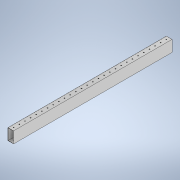
# Autodesk Inventor part: 28in OChannel 1x2
Saved by Autodesk Inventor 2020 (Build 240168000, 168)
## iProperties
Created: 2021-02-04
Part Number: 28in OChannel 1x2
Material: Aluminum 6061-AHC
Document SubType Name: Modeling
Designer: sidsa
Density: 2.7 g/cm^3
Appearance: Aluminum - Dark
Author: sidsa
Autodesk Inventor part; units mm, degrees
ref_plane "YZ Plane" through (0, 0, 0) normal (1, 0, 0) x (0, 1, 0)
ref_plane "XZ Plane" through (0, 0, 0) normal (0, 1, 0) x (-1, 0, 0)
ref_plane "XY Plane" through (0, 0, 0) normal (0, 0, 1) x (1, 0, 0)
sketch "Sketch1" plane through (0, 0, 0) normal (0, 0, 1) x (1, 0, 0)
  line L0 (0, 0) -> (25.4, 0)
  line L1 (25.4, 0) -> (25.4, 50.8)
  line L2 (25.4, 50.8) -> (0, 50.8)
  line L3 (0, 50.8) -> (0, 0)
  line L4 (24.384, 49.784) -> (24.384, 1.016)
  line L5 (24.384, 1.016) -> (1.016, 1.016)
  line L6 (1.016, 1.016) -> (1.016, 49.784)
  line L7 (1.016, 49.784) -> (24.384, 49.784)
  dimension "d0" = 25.4
  dimension "d1" = 50.8
  dimension "d2" = 1.016
  constraints: 16 end point, 4 parallel, 2 perpendicular, 1 horizontal, 3 other
  measures "d0" distance of L2.end L1.end
  measures "d1" distance of L0.end L1.end
  measures "d2" distance between parallel lines of L1 L4
extrude "Extrusion1" add sketch "Sketch1" along normal blind 711.2
sketch "Sketch2" plane through (0, 50.8, 0) normal (0, 1, 0) x (1, 0, 0)
  circle A0 centre (12.7, -12.7) radius 1.9844
  line L0 (25.4, 0) -> (0, 0) projected
  line L1 (25.4, 0) -> (25.4, -711.2) projected
  circle A1 centre (12.7, -38.1) radius 1.9844
  circle A2 centre (12.7, -63.5) radius 1.9844
  circle A3 centre (12.7, -88.9) radius 1.9844
  circle A4 centre (12.7, -114.3) radius 1.9844
  circle A5 centre (12.7, -139.7) radius 1.9844
  circle A6 centre (12.7, -165.1) radius 1.9844
  circle A7 centre (12.7, -190.5) radius 1.9844
  circle A8 centre (12.7, -215.9) radius 1.9844
  circle A9 centre (12.7, -241.3) radius 1.9844
  circle A10 centre (12.7, -266.7) radius 1.9844
  circle A11 centre (12.7, -292.1) radius 1.9844
  circle A12 centre (12.7, -317.5) radius 1.9844
  circle A13 centre (12.7, -342.9) radius 1.9844
  circle A14 centre (12.7, -368.3) radius 1.9844
  circle A15 centre (12.7, -393.7) radius 1.9844
  circle A16 centre (12.7, -419.1) radius 1.9844
  circle A17 centre (12.7, -444.5) radius 1.9844
  circle A18 centre (12.7, -469.9) radius 1.9844
  circle A19 centre (12.7, -495.3) radius 1.9844
  circle A20 centre (12.7, -520.7) radius 1.9844
  circle A21 centre (12.7, -546.1) radius 1.9844
  circle A22 centre (12.7, -571.5) radius 1.9844
  circle A23 centre (12.7, -596.9) radius 1.9844
  circle A24 centre (12.7, -622.3) radius 1.9844
  circle A25 centre (12.7, -647.7) radius 1.9844
  circle A26 centre (12.7, -673.1) radius 1.9844
  circle A27 centre (12.7, -698.5) radius 1.9844
  circle A28 centre (12.7, -723.9) radius 1.9844
  dimension "d5" = 3.9688
  dimension "d6" = 12.7
  dimension "d7" = 12.7
  dimension "d10" = 25.4
  constraints: 29 centre point, 1 vertical, 56 other
  measures "d5" diameter of A0
  measures "d6" distance from line of L0 A0.centre
  measures "d7" distance from line of L1 A0.centre
  measures "d10" distance of A0.centre A1.centre
extrude "Extrusion2" cut sketch "Sketch2" against normal blind 76.2
body "Solid1"
